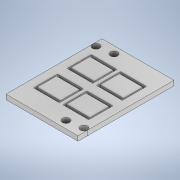
# Autodesk Inventor part: Maska2
Saved by Autodesk Inventor 2021 (Build 250183000, 183)
## iProperties
Created: 2021-04-28
Part Number: Maska2
Material: Aluminium 6061
Document SubType Name: Modeling
Designer: DESKTOP-12
Density: 2.7 g/cm^3
Appearance: Aluminium — polerowane
Author: DESKTOP-12
Autodesk Inventor part; units mm, degrees
ref_plane "YZ Plane" through (0, 0, 0) normal (1, 0, 0) x (0, 1, 0)
ref_plane "XZ Plane" through (0, 0, 0) normal (0, 1, 0) x (-1, 0, 0)
ref_plane "XY Plane" through (0, 0, 0) normal (0, 0, 1) x (1, 0, 0)
sketch "Szkic1" plane through (0, 0, 0) normal (0, 1, 0) x (-1, 0, 0)
  line L0 (0, 0) -> (30, 0)
  line L1 (30, 0) -> (30, -40)
  line L2 (30, -40) -> (0, -40)
  line L3 (0, -40) -> (0, 0)
  line L4 (3.5, -8) -> (3.5, -18)
  line L5 (3.5, -18) -> (13.5, -18)
  line L6 (13.5, -18) -> (13.5, -17)
  line L7 (13.5, -17) -> (4, -17)
  line L8 (4, -17) -> (4, -8)
  line L9 (4, -8) -> (3.5, -8)
  line L10 (4.25, -8) -> (4.25, -9)
  line L11 (14.25, -8) -> (4.25, -8)
  line L12 (4.25, -9) -> (13.75, -9)
  line L13 (14.25, -18) -> (14.25, -8)
  line L14 (13.75, -9) -> (13.75, -18)
  line L15 (13.75, -18) -> (14.25, -18)
  line L16 (15.75, -8) -> (15.75, -18)
  line L17 (15.75, -18) -> (25.75, -18)
  line L18 (25.75, -18) -> (25.75, -17)
  line L19 (25.75, -17) -> (16.25, -17)
  line L20 (16.25, -17) -> (16.25, -8)
  line L21 (16.25, -8) -> (15.75, -8)
  line L22 (16.5, -8) -> (16.5, -9)
  line L23 (26.5, -8) -> (16.5, -8)
  line L24 (16.5, -9) -> (26, -9)
  line L25 (26.5, -18) -> (26.5, -8)
  line L26 (26, -9) -> (26, -18)
  line L27 (26, -18) -> (26.5, -18)
  line L28 (3.5, -22) -> (3.5, -32)
  line L29 (3.5, -32) -> (13.5, -32)
  line L30 (13.5, -32) -> (13.5, -31)
  line L31 (13.5, -31) -> (4, -31)
  line L32 (4, -31) -> (4, -22)
  line L33 (4, -22) -> (3.5, -22)
  line L34 (4.25, -22) -> (4.25, -23)
  line L35 (14.25, -22) -> (4.25, -22)
  line L36 (4.25, -23) -> (13.75, -23)
  line L37 (14.25, -32) -> (14.25, -22)
  line L38 (13.75, -23) -> (13.75, -32)
  line L39 (13.75, -32) -> (14.25, -32)
  line L40 (26, -32) -> (26.5, -32)
  line L41 (26.5, -32) -> (26.5, -22)
  line L42 (26, -23) -> (26, -32)
  line L43 (25.75, -32) -> (25.75, -31)
  line L44 (25.75, -31) -> (16.25, -31)
  line L45 (15.75, -32) -> (25.75, -32)
  line L46 (16.5, -23) -> (26, -23)
  line L47 (26.5, -22) -> (16.5, -22)
  line L48 (16.5, -22) -> (16.5, -23)
  line L49 (16.25, -31) -> (16.25, -22)
  line L50 (16.25, -22) -> (15.75, -22)
  line L51 (15.75, -22) -> (15.75, -32)
  circle A0 centre (8, -3) radius 1.5
  circle A1 centre (1.5, -4) radius 1.5
  circle A2 centre (22, -37) radius 1.5
  circle A3 centre (28.5, -36) radius 1.5
  point P0 (15, -20)
  point P1 (0, -4)
  point P2 (30, -36)
  dimension "d10" = 360
  dimension "d0" = 30
  dimension "d1" = 40
  dimension "d2" = 10
  dimension "d4" = 1
  dimension "d5" = 9.5
  dimension "d6" = 0.5
  dimension "d7" = 8
  dimension "d12" = 0.25
  dimension "d41" = 3.5
  dimension "d42" = 10
  dimension "d50" = 3.5
  dimension "d51" = 10
  dimension "d59" = 8
  dimension "d60" = 8
  dimension "d61" = 8
  dimension "d62" = 10
  dimension "d63" = 1.5
  dimension "d64" = 0.5
  dimension "d65" = 0.25
  dimension "d66" = 3
  dimension "d67" = 8
  dimension "d68" = 3
  dimension "d69" = 4
  dimension "d70" = 1.5
  dimension "d71" = 3
  dimension "d74" = 360
  constraints: 104 end point, 21 perpendicular, 4 centre point, 4 vertical, 2 coincident, 2 parallel, 1 horizontal, 9 other
  measures "d0" distance of L1.end L2.end
  measures "d1" distance of L2.end L0.start
  measures "d2" distance of L4.start L4.end
  measures "d4" distance of L5.end L6.end
  measures "d5" distance of L6.end L7.end
  measures "d6" distance of L8.end L4.start
  measures "d7" distance from line of L4.start L0
  measures "d12" distance between parallel lines of L8 L10
  measures "d41" distance from line of L3 L4.start
  measures "d42" distance of L10.start L11.start
  measures "d50" distance from line of L25.end L1
  measures "d51" distance of L33.end L29.start
  measures "d59" distance from line of L2 L29.start
  measures "d60" distance from line of L2 L40.end
  measures "d61" distance between parallel lines of L2 L45
  measures "d62" distance of L29.end L29.start
  measures "d63" distance of L51.end L39.end
  measures "d64" distance of L39.end L38.end
  measures "d65" distance of L29.end L38.end
  measures "d66" distance from line of L0 point (8, -3)
  measures "d67" distance from line of L3 point (8, -3)
  measures "d68" diameter of A0
  measures "d69" distance from line of L0 point (1.5, -4)
  measures "d70" distance from line of L3 point (1.5, -4)
  measures "d71" diameter of A1
extrude "Wyciągnięcie proste1" add sketch "Szkic1" along normal blind 2
